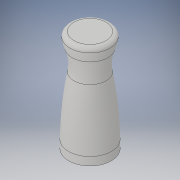
# Autodesk Inventor part: Cutting Template
Saved by Autodesk Inventor 2019 (Build 230136000, 136)
## iProperties
Created: 2019-02-23
Part Number: Cutting Template
Material: Generic
Document SubType Name: Modeling
Designer: Kepler
Density: 1 g/cm^3
Appearance: Default
Author: Kepler
Autodesk Inventor part; units mm, degrees
ref_plane "YZ Plane" through (0, 0, 0) normal (1, 0, 0) x (0, 1, 0)
ref_plane "XZ Plane" through (0, 0, 0) normal (0, 1, 0) x (-1, 0, 0)
ref_plane "XY Plane" through (0, 0, 0) normal (0, 0, 1) x (1, 0, 0)
sketch "Sketch1" plane through (0, 0, 0) normal (0, 0, 1) x (1, 0, 0)
  line L0 (0, 0) -> (10.5, 0)
  line L1 (10.5, 0) -> (10.5, 4)
  line L2 (0, 0) -> (0, 50)
  line L3 (0, 50) -> (10, 50)
  arc A0 (8.7939, 43.1596) -> (10, 50) centre (-10, 50) ccw
  line L4 (-10, 50) -> (8.7939, 43.1596) construction
  line L5 (-10, 50) -> (10, 50) construction
  arc A1 (8.7939, 43.1596) -> (7.8915, 32.8462) centre (27.5877, 36.3192) ccw
  line L6 (27.5877, 36.3192) -> (7.8915, 32.8462) construction
  line L7 (27.5877, 36.3192) -> (8.7939, 43.1596) construction
  arc A2 (10.5, 4) -> (7.8915, 32.8462) centre (-161.3854, 2.9981) ccw
  dimension "d1" = 10.5
  dimension "d2" = 4
  dimension "d3" = 50
  dimension "d4" = 10
  dimension "d5" = 20
  dimension "d6" = 10
  dimension "d8" = 6.8404
  dimension "d9" = 30
  dimension "d10" = 20
  dimension "d12" = 20
  dimension "d13" = 0
  constraints: 16 end point, 6 point on circle, 3 centre point, 2 perpendicular, 2 tangent, 1 horizontal, 1 vertical
  measures "d1" distance of L0.start L0.end
  measures "d2" distance of L0.end L1.end
  measures "d3" distance of L0.start L2.end
  measures "d4" distance of L2.end L3.end
  measures "d5" angle of L4 L5
  measures "d6" distance from line of L4.start L2
  measures "d8" distance from line of L4.end L3
  measures "d9" angle of L7 L6
  measures "d10" distance of L4.start L4.end
  measures "d12" distance of L6.start L4.end
  measures "d13" distance from line of L4.start L3
revolve "Revolution1" add sketch "Sketch1" angle 360 about axis through (0, 0, 0) along (0, 1, 0)
fillet "Fillet1" radius 2 1 edges at (-10, 50, 0)
body "Solid1"
